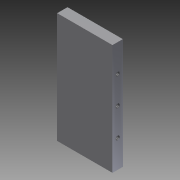
# Autodesk Inventor part: plate_connect_block
Saved by Autodesk Inventor 2012 (Build 160160000, 160)
## iProperties
Created: 2012-01-29
Part Number: plate_connect_block
Material: Default
Document SubType Name: Modeling
Designer: Antonella Wilby
Density: 1 g/cm^3
Author: Antonella Wilby
Autodesk Inventor part; units mm, degrees
ref_plane "YZ Plane" through (0, 0, 0) normal (1, 0, 0) x (0, 1, 0)
ref_plane "XZ Plane" through (0, 0, 0) normal (0, 1, 0) x (-1, 0, 0)
ref_plane "XY Plane" through (0, 0, 0) normal (0, 0, 1) x (1, 0, 0)
sketch "Sketch1" plane through (0, 0, 0) normal (0, 0, 1) x (1, 0, 0)
  line L0 (-35.56, 0) -> (35.56, 0) projected
  line L1 (0, -71.12) -> (0, 71.12) projected
  line L2 (-25.4, 50.8) -> (25.4, 50.8)
  line L3 (25.4, 50.8) -> (25.4, -50.8)
  line L4 (25.4, -50.8) -> (-25.4, -50.8)
  line L5 (-25.4, -50.8) -> (-25.4, 50.8)
  point P0 (0, 0)
  point P1 (-25.4, 0)
  point P2 (0, 50.8)
  dimension "d0" = 101.6
  dimension "d1" = 50.8
  constraints: 8 end point, 2 midpoint, 2 parallel, 1 horizontal, 1 horizontal alignment, 1 perpendicular, 1 vertical alignment
  measures "d0" distance of L4.end L2.start
  measures "d1" distance of L2.start L2.end
extrude "Extrusion1" add sketch "Sketch1" along normal mid plane 9.525
sketch "Sketch2" plane through (25.4, -50.8, 4.7625) normal (1, 0, 0) x (0, 0, -1)
  point P0 (4.7625, 50.8)
  point P1 (4.7625, 76.2)
  point P2 (4.7625, 50.8)
  point P3 (4.7625, 25.4)
  dimension "d4" = 25.4
  dimension "d5" = 25.4
  constraints: 2 vertical alignment, 1 coincident
  measures "d4" distance of point (4.763, 50.8) point (4.763, 25.4)
  measures "d5" distance of point (4.763, 76.2) point (4.763, 50.8)
hole "Hole1" at (25.4, 25.4, 0) at (25.4, 0, 0) at (25.4, -25.4, 0) direction (-1, 0, 0) diameter 3.683 depth 19.05 tip angle 118 thread size "10-24 UNC" class "2B" standard "ANSI Unified Screw Threads"
mirror "Mirror1" about plane through (0, 0, 0) normal (1, 0, 0) of "Hole1"
body "Solid1"
